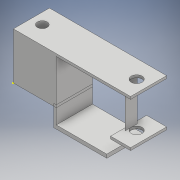
# Autodesk Inventor part: finge
Saved by Autodesk Inventor 2017 (Build 210142000, 142)
## iProperties
Created: 2016-12-21
Part Number: finge
Material: Generic
Document SubType Name: Modeling
Designer: Samanth
Density: 1 g/cm^3
Appearance: Default
Author: Samanth
Autodesk Inventor part; units mm, degrees
ref_plane "YZ Plane" through (0, 0, 0) normal (1, 0, 0) x (0, 1, 0)
ref_plane "XZ Plane" through (0, 0, 0) normal (0, 1, 0) x (-1, 0, 0)
ref_plane "XY Plane" through (0, 0, 0) normal (0, 0, 1) x (1, 0, 0)
sketch "Sketch1" plane through (0, 0, 0) normal (0, 0, 1) x (1, 0, 0)
  line L0 (0, 0) -> (65, 0)
  line L1 (0, 0) -> (0, 10)
  line L2 (0, 10) -> (65, 10)
  line L3 (65, 10) -> (65, -10)
  line L4 (65, -10) -> (0, -10)
  line L5 (0, -10) -> (0, 0)
  dimension "d0" = 65
  dimension "d1" = 10
  dimension "d2" = 65
  dimension "d3" = 20
  constraints: 12 end point, 3 perpendicular, 1 collinear, 1 horizontal, 1 point on line, 1 vertical
  measures "d0" distance of L0.start L0.end
  measures "d1" distance of L0.start L1.end
  measures "d2" distance of L1.end L2.end
  measures "d3" distance of L2.end L3.end
extrude "Extrusion1" add sketch "Sketch1" along normal blind 26
sketch "Sketch2" plane through (0, 0, 26) normal (0, 0, 1) x (1, 0, 0)
  circle A0 centre (6.028, 0) radius 2.7
  circle A1 centre (58.4004, 0) radius 2.7
  point P0 (0, 0)
  dimension "d6" = 5.4
  dimension "d7" = 5.4
  constraints: 2 centre point
  measures "d6" diameter of A0
  measures "d7" diameter of A1
extrude "Extrusion2" cut sketch "Sketch2" against normal blind 26
sketch "Sketch3" plane through (0, 10, 0) normal (0, 1, 0) x (1, 0, 0)
  line L0 (65, 0) -> (65, -26) projected
  line L1 (65, -13) -> (65, -1.4)
  line L2 (65, -1.4) -> (65, -24.6)
  line L3 (65, -24.6) -> (23.8068, -24.6)
  line L4 (23.8068, -24.6) -> (23.8068, -1.4)
  line L5 (23.8068, -1.4) -> (65, -1.4)
  point P0 (0, 0)
  dimension "d10" = 11.6
  dimension "d11" = 23.2
  constraints: 10 end point, 3 perpendicular, 2 point on line, 1 midpoint
  measures "d10" distance of L1.start L1.end
  measures "d11" distance of L1.end L2.end
extrude "Extrusion3" cut sketch "Sketch3" against normal blind 20
sketch "Sketch4" plane through (0, -10, 0) normal (0, -1, 0) x (1, 0, 0)
  point P0 (0, 0)
sketch "Sketch8" plane through (65, 10, 24.6) normal (0, 0, -1) x (-1, 0, 0)
  circle A0 centre (6.5996, -10) radius 2.7 projected
  circle A1 centre (6.5996, -10) radius 3
  circle A2 centre (6.5996, -10) radius 3
  point P0 (65, -10)
  dimension "d22" = 6
  dimension "d23" = 6
  constraints: 2 centre point, 2 coincident
  measures "d22" diameter of A1
  measures "d23" diameter of A2
extrude "Extrusion7" cut sketch "Sketch8" along normal mid plane 60 contours A0 | A1
sketch "Sketch9" plane through (0, 10, 0) normal (0, 1, 0) x (1, 0, 0)
  line L0 (65, -1.4) -> (23.8068, -1.4) projected
  line L1 (23.8068, -1.4) -> (23.8068, 8.27)
  line L2 (23.8068, 8.27) -> (51.8068, 8.27)
  line L3 (51.8068, 8.27) -> (51.8068, 10.27)
  line L4 (51.8068, 10.27) -> (22.4262, 10.27)
  line L5 (22.4262, 10.27) -> (22.4262, -1.4)
  line L6 (22.4262, -1.4) -> (23.8068, -1.4)
  point P0 (0, 0)
  dimension "d26" = 9.67
  dimension "d27" = 28
  dimension "d28" = 2
  constraints: 12 end point, 4 perpendicular, 1 horizontal, 1 vertical
  measures "d26" distance of L0.end L1.end
  measures "d27" distance of L1.end L2.end
  measures "d28" distance of L2.end L3.end
extrude "Extrusion8" add sketch "Sketch9" against normal blind 20 separate body
sketch "Sketch10" plane through (23.8068, 10, 1.4) normal (0, 0, 1) x (1, 0, 0)
  circle A0 centre (34.5936, -10) radius 3 projected
  circle A1 centre (34.5936, -10) radius 4.5
  circle A2 centre (34.5936, -10) radius 3 projected
  circle A3 centre (34.5936, -10) radius 3
  line L0 (31.5917, -6.6476) -> (31.5917, -13.3524)
  line L1 (28, 0) -> (28, -20) projected
  point P0 (-23.8068, -10)
  dimension "d31" = 9
  constraints: 2 centre point, 2 coincident, 2 end point, 2 point on circle, 1 parallel
  measures "d31" diameter of A1
extrude "Extrusion9" add sketch "Sketch10" along normal blind 23.75 contours L0 A1 picked at (31.1031, -9.8203) bodies 1
sketch "Sketch11" plane through (0, 10, 0) normal (0, 1, 0) x (1, 0, 0)
  line L0 (65, -1.4) -> (23.8068, -1.4) projected
  line L1 (23.8068, -1.4) -> (53.9004, -1.4)
  line L2 (53.9004, -1.4) -> (53.9004, 0)
  line L3 (53.9004, 0) -> (23.8068, 0)
  line L4 (23.8068, 0) -> (23.8068, -1.4)
  point P0 (0, 0)
  constraints: 8 end point, 2 parallel, 1 horizontal, 1 perpendicular
extrude "Extrusion10" cut sketch "Sketch11" against normal blind 23.75 bodies 1
body "Solid1"
body "Solid2"
